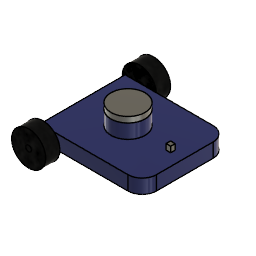
squarobot_mini (Autodesk Fusion 360 design; units mm, degrees)
Autodesk Fusion 360 part; units mm, degrees
sketch "Sketch1" plane through (0, 0, 0) normal (0, 0, 1) x (1, 0, 0)
  line L0 (100, -75) -> (-100, -75)
  line L1 (-100, -75) -> (-100, 75)
  line L2 (-100, 75) -> (100, 75)
  line L3 (100, 75) -> (100, -75)
  line L4 (100, -75) -> (-100, 75) construction
  line L5 (-100, -75) -> (100, 75) construction
  dimension "d1" = 200
  dimension "d2" = 150
  constraint horizontal L0
  constraint perpendicular L0 L1
  constraint parallel L0 L2
  constraint parallel L1 L3
  constraint coincident L4 origin
  constraint coincident L5 origin
  measures "d1" distance of L1.end L2.end
  measures "d2" distance of L0.end L1.end
extrude "Extrude1" add sketch "Sketch1" along normal blind 25 makes body 1
sketch "Sketch2" plane through (0, -75, 0) normal (0, -1, 0) x (1, 0, 0)
  line L0 (-100, 0) -> (100, 0)
  line L1 (100, 0) -> (100, 25)
  line L2 (100, 25) -> (-100, 25)
  line L3 (-100, 25) -> (-100, 0)
  line L4 (-100, 12.5) -> (-65, 12.5)
  circle A0 centre (-65, 12.5) radius 5
  dimension "d5" = 35
  dimension "d6" = 10
  constraint midpoint L3 L4.start
  constraint perpendicular L3 L4
  constraint coincident L4.end A0.centre
  measures "d5" distance of L4.start L4.end
  measures "d6" diameter of A0
extrude "Extrude2" add sketch "Sketch2" along normal blind 10 contours A0 bodies 1
sketch "Sketch3" plane through (0, -85, 0) normal (0, -1, 0) x (1, 0, 0)
  circle A0 centre (-65, 12.5) radius 5
  circle A1 centre (-65, 12.5) radius 30
  dimension "d9" = 60
  constraint concentric A0 A1
  measures "d9" diameter of A1
extrude "Extrude3" add sketch "Sketch3" along normal blind 25 separate body makes body 2
mirror "Mirror1" about plane through (0, 0, 0) normal (0, 1, 0) of "Extrude2", "Extrude3" makes body 3
ref_plane "WorkPlane1" through (-65, 100.2089, -17.5) normal (0, 0, -1) x (-1, 0, 0)
move_body "Move1" bodies 1 2 3 to x (1, 0, 0) y (0, 1, 0) z (0, 0, 1) at (0, 0, 17.5)
sketch "Sketch4" plane through (0, 0, 17.5) normal (0, 0, -1) x (1, 0, 0)
  line L0 (-100, -75) -> (100, -75)
  line L1 (100, -75) -> (100, 75)
  line L2 (100, 75) -> (-100, 75)
  line L3 (-100, 75) -> (-100, -75)
  line L4 (100, 0) -> (70, 0)
  circle A0 centre (70, 0) radius 15
  dimension "d15" = 30
  dimension "d16" = 30
  constraint midpoint L1 L4.start
  constraint perpendicular L1 L4
  constraint coincident L4.end A0.centre
  measures "d15" distance of L4.start L4.end
  measures "d16" diameter of A0
extrude "Extrude4" add sketch "Sketch4" along normal blind 17.5 separate body contours A0 makes body 4
fillet "Fillet1" radius 15 1 faces at (69.464, -3.9092, 0) on bodies 4
sketch "Sketch5" plane through (0, 0, 42.5) normal (0, 0, 1) x (-1, 0, 0)
  line L0 (-100, -75) -> (100, -75)
  line L1 (100, -75) -> (100, 75)
  line L2 (100, 75) -> (-100, 75)
  line L3 (-100, 75) -> (-100, -75)
  circle A0 centre (0, 0) radius 30
  dimension "d21" = 60
  constraint coincident A0.centre origin
  measures "d21" diameter of A0
extrude "Extrude5" add sketch "Sketch5" along normal blind 25 contours A0 bodies 1
sketch "Sketch6" plane through (0, 0, 67.5) normal (0, 0, 1) x (-1, 0, 0)
  circle A0 centre (0, 0) radius 30
extrude "Extrude6" add sketch "Sketch6" along normal blind 10 separate body makes body 5
chamfer "Chamfer1" distance 20 angle 45 1 edges at (-100, 0, 42.5) on bodies 1
fillet "Fillet2" radius 25 1 edges at (100, -75, 30) on bodies 1
fillet "Fillet3" radius 25 1 edges at (100, 75, 30) on bodies 1
copy_body "Body->Comp1" bodies 1 removing the originals makes body 6 in component "base_link"
copy_body "Body->Comp2" bodies 2 removing the originals makes body 7 in component "right_wheel"
copy_body "Body->Comp3" bodies 3 removing the originals makes body 8 in component "left_wheel"
copy_body "Body->Comp4" bodies 4 removing the originals makes body 9 in component "caster"
copy_body "Body->Comp5" bodies 5 removing the originals makes body 10 in component "lidar"
sketch "Sketch7" plane through (0, 0, 42.5) normal (0, 0, 1) x (-1, 0, 0)
  arc A0 (-100, -50) -> (-75, -75) centre (-75, -50) ccw
  line L0 (-75, -75) -> (80, -75)
  line L1 (80, -75) -> (80, 75)
  line L2 (80, 75) -> (-75, 75)
  arc A1 (-75, 75) -> (-100, 50) centre (-75, 50) ccw
  line L3 (-100, 50) -> (-100, -50)
  circle A2 centre (0, 0) radius 30
  line L4 (-84.0825, 3.9881) -> (-75.9175, 3.9881)
  line L5 (-75.9175, 3.9881) -> (-75.9175, -3.9881)
  line L6 (-75.9175, -3.9881) -> (-84.0825, -3.9881)
  line L7 (-84.0825, -3.9881) -> (-84.0825, 3.9881)
  line L8 (-84.0825, 3.9881) -> (-75.9175, -3.9881) construction
  line L9 (-75.9175, 3.9881) -> (-84.0825, -3.9881) construction
  point P0 (-80, 0)
  constraint horizontal L4
  constraint perpendicular L4 L5
  constraint parallel L4 L6
  constraint parallel L5 L7
  constraint coincident L8 P0
  constraint coincident L9 P0
extrude "Extrude1'" add sketch "Sketch7" along normal blind 10 separate body contours L4 L5 L6 L7 makes body 11 in component "camera"
component "base_link" placed x (1, 0, 0) y (0, 1, 0) z (0, 0, 1) at (0, 0, 0)
component "right_wheel" placed x (1, 0, 0) y (0, 1, 0) z (0, 0, 1) at (0, 0, 0)
component "left_wheel" placed x (1, 0, 0) y (0, 1, 0) z (0, 0, 1) at (0, 0, 0)
component "caster" placed x (1, 0, 0) y (0, 1, 0) z (0, 0, 1) at (0, 0, 0)
component "lidar" placed x (1, 0, 0) y (0, 1, 0) z (0, 0, 1) at (0, 0, 0)
component "camera" placed x (1, 0, 0) y (0, 1, 0) z (0, 0, 1) at (-5, 0, 0)
named bodies: "base_link", "right_wheel", "left_wheel", "caster", "lidar"
